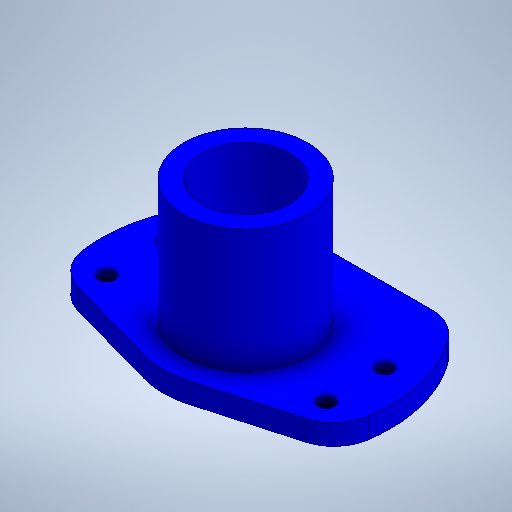
# Autodesk Inventor part: SyringeHolder
Saved by Autodesk Inventor 2025.2 (Build 292293000, 293)
## iProperties
Created: 2025-05-31
Part Number: SyringeHolder
Material: Generic
Document SubType Name: Modeling
Designer: Simon
Density: 1 g/cm^3
Appearance: Default(1)
Author: Simon
Autodesk Inventor part; units mm, degrees
ref_plane "YZ Plane" through (0, 0, 0) normal (1, 0, 0) x (0, 1, 0)
ref_plane "XZ Plane" through (0, 0, 0) normal (0, 1, 0) x (-1, 0, 0)
ref_plane "XY Plane" through (0, 0, 0) normal (0, 0, 1) x (1, 0, 0)
sketch "Sketch1" plane through (0, 0, 0) normal (0, 1, 0) x (-1, 0, 0)
  circle A0 centre (0, 0) radius 35
  circle A1 centre (0, 0) radius 10.7
  line L0 (0, 0) -> (0, -48)
  line L1 (60, -48) -> (-60, -48)
  circle A2 centre (-60, -48) radius 50
  circle A3 centre (60, -48) radius 50
  circle A4 centre (0, 0) radius 20
  line L2 (73.5118, 0.1397) -> (5.4047, 19.2559)
  line L3 (-73.5118, 0.1397) -> (-5.4047, 19.2559)
  line L4 (0, 0) -> (0, -25)
  line L5 (24.4949, -25) -> (-24.4949, -25)
  circle A5 centre (0, 0) radius 27.5
  line L6 (0, 0) -> (-26.563, 7.1175)
  line L7 (0, 0) -> (27.5, 0) construction
  line L8 (0, 0) -> (-26.563, -7.1175)
  line L9 (0, 0) -> (26.563, 7.1175)
  line L10 (0, 0) -> (26.563, -7.1175)
  point P0 (33.0589, 11.494)
  point P1 (-33.0589, 11.494)
  dimension "d0" = 70
  dimension "d10" = 100
  dimension "d11" = 100
  dimension "d1" = 21.4
  dimension "d8" = 48
  dimension "d9" = 120
  dimension "d12" = 40
  dimension "d13" = 25
  dimension "d18" = 55
  dimension "d19" = 165
  constraints: 22 end point, 6 coincident, 6 point on circle, 3 centre point, 2 horizontal, 2 midpoint, 2 tangent, 1 equal length, 1 perpendicular, 1 point on line, 1 vertical, 11 other
  measures "d1" diameter of A1
  measures "d8" distance of L0.start L0.end
  measures "d9" distance of L1.start L1.end
  measures "d12" diameter of A4
  measures "d13" distance of L4.start L4.end
  measures "d18" diameter of A5
  measures "d19" angle of L7 L6
extrude "Extrusion1" add sketch "Sketch1" along normal blind 5 contours A0 A3 A5 L2 | A0 L5 A3 A5 | L3 A5 A2 A0 | A5 L9 A4 L2 | A5 A3 | A3 A5 L5 L0 A4 L10 | A2 A5 L5 A0 | L3 A4 L6 A5 | A4 L9 A1 L6 | A5 L10 A4 L9 | L5 A5 A3 | A5 L8 A4 L0 L5 A2 | A2 A5 | L6 A4 L8 A5 | A4 L10 A1 L9 | A4 L0 A1 L10 | A2 A5 L5 | L6 A1 L8 A4 | A4 L8 A1 L0
fillet "Fillet1" radius 10 4 edges at (33.0589, 2.5, 11.494) (-33.0589, 2.5, 11.494) (24.4949, 2.5, -25) (-24.4949, 2.5, -25)
sketch "Sketch3" plane through (0, 5, 0) normal (0, 1, 0) x (1, 0, 0)
  circle A0 centre (0, 0) radius 10.7
  circle A1 centre (0, 0) radius 15
  dimension "d15" = 30
  constraints: 2 centre point, 2 coincident
  measures "d15" diameter of A1
extrude "Extrusion3" add sketch "Sketch3" along normal blind 30
hole "Hole1" at (26.563, 0, 7.1175) at (26.563, 0, -7.1175) at (-26.563, 0, 7.1175) at (-26.563, 0, -7.1175) direction (0, 1, 0) diameter 4 end through all
body "Solid1"
